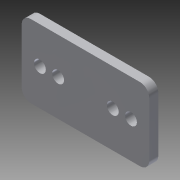
# Autodesk Inventor part: Bearing Mount Spacer 1-8 in
Saved by Autodesk Inventor 2014 (Build 180170000, 170)
## iProperties
Created: 2014-01-16
Part Number: Bearing Mount Spacer 1-8 in
Material: Aluminum 6061
Document SubType Name: Modeling
Designer: Michael
Density: 2.71 g/cm^3
Appearance: Aluminum - Flat
Author: Michael
Autodesk Inventor part; units mm, degrees
ref_plane "YZ Plane" through (0, 0, 0) normal (1, 0, 0) x (0, 1, 0)
ref_plane "XZ Plane" through (0, 0, 0) normal (0, 1, 0) x (-1, 0, 0)
ref_plane "XY Plane" through (0, 0, 0) normal (0, 0, 1) x (1, 0, 0)
sketch "Sketch1" plane through (0, 0, 0) normal (0, 0, 1) x (1, 0, 0)
  line L0 (3.175, 0) -> (41.275, 0)
  line L1 (44.45, 3.175) -> (44.45, 22.225)
  line L2 (41.275, 25.4) -> (3.175, 25.4)
  line L3 (0, 22.225) -> (0, 3.175)
  circle A0 centre (6.35, 12.7) radius 2.0701
  circle A1 centre (31.75, 12.7) radius 2.0701
  circle A2 centre (12.7, 12.7) radius 2.0701
  line L4 (0, 12.7) -> (44.45, 12.7) construction
  circle A3 centre (38.1, 12.7) radius 2.0701
  arc A4 (3.175, 25.4) -> (0, 22.225) centre (3.175, 22.225) ccw
  arc A5 (44.45, 22.225) -> (41.275, 25.4) centre (41.275, 22.225) ccw
  arc A6 (41.275, 0) -> (44.45, 3.175) centre (41.275, 3.175) ccw
  arc A7 (0, 3.175) -> (3.175, 0) centre (3.175, 3.175) ccw
  point P0 (0, 0)
  point P1 (44.45, 25.4)
  point P2 (44.45, 0)
  point P3 (0, 25.4)
  dimension "d0" = 44.45
  dimension "d1" = 25.4
  dimension "d2" = 4.1402
  dimension "d3" = 6.35
  dimension "d7" = 25.4
  dimension "d12" = 6.35
  dimension "d15" = 25.4
  dimension "d20" = 3.175
  constraints: 10 end point, 10 point on line, 8 centre point, 8 point on circle, 8 tangent, 4 equal radius, 3 horizontal, 2 midpoint, 2 parallel, 1 perpendicular, 4 other
  measures "d0" distance of point (0, 25.4) point (44.45, 25.4)
  measures "d1" distance of point (44.45, 25.4) point (44.45, 0)
  measures "d2" diameter of A0
  measures "d3" distance from line of L3 A0.centre
  measures "d7" distance of A0.centre A1.centre
  measures "d12" distance of A0.centre A2.centre
  measures "d15" distance of A2.centre A3.centre
  measures "d20" radius of A4
extrude "Extrusion1" add sketch "Sketch1" along normal blind 3.175
body "Solid1"
